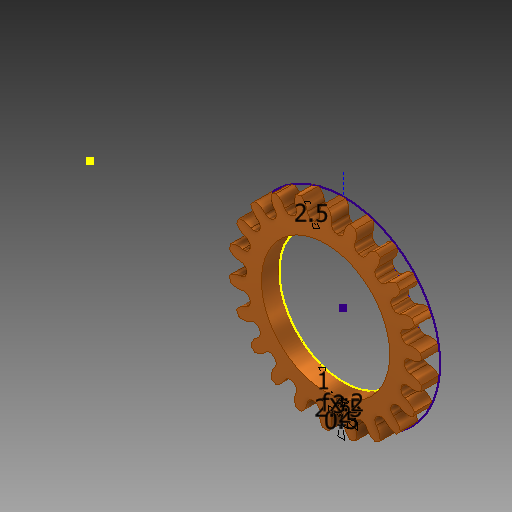
# Autodesk Inventor part: CreeGear
Saved by Autodesk Inventor 2017 (Build 210142000, 142)
## iProperties
Created: 2017-02-15
Part Number: CreeGear
Material: Gold
Document SubType Name: Modeling
Designer: Moonlight.Admin
Density: 19.3 g/cm^3
Appearance: Metal 1600F Hot
Author: Moonlight.Admin
Autodesk Inventor part; units mm, degrees
ref_plane "YZ Plane" through (0, 0, 0) normal (1, 0, 0) x (0, 1, 0)
ref_plane "XZ Plane" through (0, 0, 0) normal (0, 1, 0) x (-1, 0, 0)
ref_plane "XY Plane" through (0, 0, 0) normal (0, 0, 1) x (1, 0, 0)
derived "CombinedHousingV2.ipt"
sketch "CreeLED" plane through (0, 0, 0) normal (0, 0, 1) x (1, 0, 0)
  line L0 (30.125, 24.13) -> (56.625, 24.13)
  line L1 (56.625, 24.13) -> (56.625, -24.13)
  line L2 (56.625, -24.13) -> (30.125, -24.13)
  line L3 (30.125, -24.13) -> (30.125, 24.13)
  circle A0 centre (43.375, 0) radius 11
  line L4 (30.125, 24.13) -> (56.625, -24.13) construction
  line L5 (25.125, 25.125) -> (25.125, -25.125) construction
  line L6 (-25.125, 25.125) -> (25.125, 25.125) construction
  circle A1 centre (43.375, 9.5) radius 3.5
  circle A2 centre (33.875, 0) radius 3.5
  circle A3 centre (52.875, 0) radius 3.5
  circle A4 centre (43.375, -9.5) radius 3.5
  circle A5 centre (37.025, 18.2562) radius 2.032
  circle A6 centre (49.725, 18.2562) radius 2.032
  circle A7 centre (49.725, -18.2563) radius 2.032
  circle A8 centre (37.025, -18.2563) radius 2.032
  point P0 (0, 0)
sketch "Sketch2" plane through (0, 0, 0) normal (0, 0, 1) x (1, 0, 0)
  circle A0 centre (43.375, 0) radius 11 projected
  arc A1 (42.875, -16.5015) -> (43.875, -16.5015) centre (43.375, -13.5435) ccw
  arc A2 (43.875, -16.5015) -> (44.375, -14.5015) centre (41.6516, -14.8832) ccw
  line L0 (42.875, -16.5015) -> (43.875, -16.5015) construction
  arc A3 (42.375, -14.5015) -> (42.875, -16.5015) centre (45.0984, -14.8832) ccw
  line L1 (42.375, -14.5015) -> (44.375, -14.5015) construction
  arc A4 (42.375, -14.5015) -> (40.3847, -14.3628) centre (41.3847, -14.3628) ccw
  arc A5 (46.3653, -14.3628) -> (44.375, -14.5015) centre (45.3653, -14.3628) ccw
  line L2 (40.3847, -14.3628) -> (40.3847, -17.0015)
  line L3 (40.3847, -17.0015) -> (46.3653, -17.0015)
  line L4 (46.3653, -17.0015) -> (46.3653, -14.3628)
  line L5 (43.375, 20.4133) -> (43.375, 12.8025) construction
  circle A6 centre (43.375, 0) radius 13.5 construction
  circle A7 centre (43.375, 0) radius 16.5435
  point P0 (0, 0)
  point P1 (43.375, -14.5015)
  point P2 (43.375, -16.5015)
  dimension "d1" = 3
  dimension "d2" = 2
  dimension "d3" = 0.5
  dimension "d4" = 1
  dimension "d5" = 2
  dimension "d6" = 2.75
  dimension "d8" = 1
  dimension "d9" = 2.5
  constraints: 13 end point, 10 point on circle, 7 centre point, 6 tangent, 3 point on line, 2 coincident, 2 equal radius, 2 midpoint, 2 parallel, 1 perpendicular, 1 vertical
  measures "d1" radius of A1
  measures "d2" distance of L1.end L1.start
  measures "d3" distance between parallel lines of L3 L0
  measures "d4" radius of A4
  measures "d5" distance between parallel lines of L0 L1
  measures "d6" radius of A3
  measures "d8" distance of L0.start L0.end
  measures "d9" radial gap between concentric circles of A6 A0
extrude "Extrusion1" add sketch "Sketch2" along normal blind 3 contours A3 A4 L2 A7 L4 A5 A2 A1 | A1 A7 L2 A4 A3 | A1 A2 A5 L4 A7
extrude "Extrusion2" cut sketch "Sketch2" along normal blind 3 contours A1 A7 L2 A4 A3 | A7 L4 L3 L2 | A1 A2 A5 L4 A7
pattern_circular "Circular Pattern1" count 22 over 360 about axis through (43.375, 0, 0) along (0, 0, 1) of "Extrusion2"
body "Solid1"
